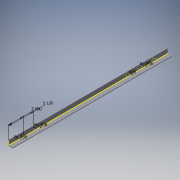
# Autodesk Inventor part: 32.25 Top L w holes
Saved by Autodesk Inventor 2016 SP2 (Build 200236200, 236)
## iProperties
Created: 2018-01-25
Part Number: 32.25 Top L w holes
Material: Generic
Document SubType Name: Modeling
Designer: CAD
Density: 1 g/cm^3
Appearance: Default
Author: CAD
Autodesk Inventor part; units mm, degrees
ref_plane "YZ Plane" through (0, 0, 0) normal (1, 0, 0) x (0, 1, 0)
ref_plane "XZ Plane" through (0, 0, 0) normal (0, 1, 0) x (-1, 0, 0)
ref_plane "XY Plane" through (0, 0, 0) normal (0, 0, 1) x (1, 0, 0)
sketch "Sketch1" plane through (0, 0, 0) normal (0, 0, 1) x (1, 0, 0)
  line L0 (0, 0) -> (-25.4, 0)
  line L1 (-25.4, 0) -> (-25.4, 25.4)
  line L2 (0, 3.175) -> (-22.225, 3.175)
  line L3 (-22.225, 3.175) -> (-22.225, 25.4)
  line L4 (-22.225, 25.4) -> (-25.4, 25.4)
  line L5 (0, 3.175) -> (0, 0)
  dimension "d0" = 25.4
  dimension "d1" = 25.4
  dimension "d2" = 3.175
  constraints: 12 end point, 3 perpendicular, 2 horizontal, 1 other
  measures "d0" distance of L0.start L0.end
  measures "d1" distance of L0.end L1.end
  measures "d2" distance between parallel lines of L0 L2
extrude "Extrusion1" add sketch "Sketch1" along normal mid plane 819.15
sketch "Sketch2" plane through (-22.225, 3.175, 409.575) normal (1, 0, 0) x (0, 0, -1)
  line L0 (0, 0) -> (819.15, 0) projected
  line L1 (0, 0) -> (0, 22.225) projected
  point P0 (409.575, -3.175)
  point P1 (76.2, 11.1125)
  point P2 (130.175, 11.1125)
  point P3 (608.8665, 11.1125)
  point P4 (739.8729, 11.1125)
  dimension "d5" = 11.1125
  dimension "d6" = 11.1125
  dimension "d7" = 11.1125
  dimension "d8" = 11.1125
  dimension "d9" = 76.2
  dimension "d10" = 130.175
  measures "d5" distance from line of L0 point (608.867, 11.112)
  measures "d6" distance from line of L0 point (739.873, 11.112)
  measures "d7" distance from line of L0 point (130.175, 11.112)
  measures "d8" distance from line of L0 point (76.2, 11.112)
  measures "d9" distance from line of L1 point (76.2, 11.112)
  measures "d10" distance from line of point (130.175, 11.112) L1
sketch "Sketch3" plane through (-22.225, 3.175, 409.575) normal (1, 0, 0) x (0, 0, -1)
  circle A0 centre (144.907, 9.779) radius 3.302 projected
  circle A1 centre (126.9411, 8.2233) radius 2.0193 projected
  circle A2 centre (73.9729, 8.2233) radius 2.4955 projected
  circle A3 centre (56.007, 9.779) radius 3.302 projected
  circle A4 centre (755.269, 9.525) radius 3.7782 projected
  circle A5 centre (737.3031, 7.9693) radius 4.7625 projected
  circle A6 centre (684.3349, 7.9693) radius 2.9083 projected
  circle A7 centre (666.369, 9.525) radius 4.572 projected
  point P0 (409.575, -3.175)
hole "Hole1" at (-22.225, 12.7, -345.694) at (-22.225, 11.1443, -327.7281) at (-22.225, 11.1443, -274.7599) at (-22.225, 12.7, -256.794) at (-22.225, 12.954, 353.568) at (-22.225, 11.3983, 335.6021) at (-22.225, 11.3983, 282.6339) at (-22.225, 12.954, 264.668) direction (-1, 0, 0) diameter 6.35 depth 25.4 tip angle 118
equation "\"d6\" = d5"
equation "\"d7\" = d5"
equation "\"d8\" = d5"
body "Solid1"
